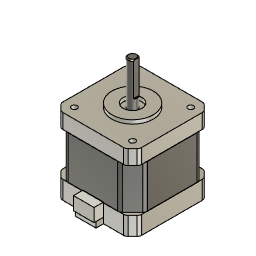
NEMA17StepperMotor (Autodesk Fusion 360 design; units mm, degrees)
Autodesk Fusion 360 part; units mm, degrees
sketch "Sketch1" plane through (0, 0, 0) normal (0, 0, 1) x (1, 0, 0)
  line L0 (-15.5, -15.5) -> (15.5, -15.5) construction
  line L1 (15.5, -15.5) -> (15.5, 15.5) construction
  line L2 (15.5, 15.5) -> (-15.5, 15.5) construction
  line L3 (-15.5, 15.5) -> (-15.5, -15.5) construction
  line L4 (0, 0) -> (0, 15.5) construction
  line L5 (0, 0) -> (15.5, 0) construction
  line L6 (-21, -21) -> (21, -21)
  line L7 (21, -21) -> (21, 21)
  line L8 (21, 21) -> (-21, 21)
  line L9 (-21, 21) -> (-21, -21)
  line L10 (-19.0919, 19.0919) -> (19.0919, -19.0919) construction
  line L11 (-21, 21) -> (21, -21) construction
  line L12 (-21, -21) -> (21, 21) construction
  line L13 (-21, 17.1838) -> (-17.1838, 21)
  line L14 (-17.1838, -21) -> (-21, -17.1838)
  line L15 (21, -17.1838) -> (17.1838, -21)
  line L16 (17.1838, 21) -> (21, 17.1838)
  dimension "d1" = 31
  dimension "d2" = 5.5
  dimension "d3" = 54
  dimension "d5" = 360
  constraint horizontal L0
  constraint vertical L1
  constraint horizontal L2
  constraint vertical L3
  constraint coincident L4.start L5.start
  constraint midpoint L1 L5.end
  constraint horizontal L5
  constraint midpoint L2 L4.end
  constraint vertical L4
  constraint equal L1 L2
  constraint coincident L4.start L10
  constraint coincident L10.end L11
  constraint coincident L10.start L11
  constraint symmetric L10.start L10.end L12
  constraint coincident L9 L13.start
  constraint coincident L8 L13.end
  constraint coincident L10.start L13
  constraint perpendicular L10 L13
  measures "d1" distance of L0.start L0.end
  measures "d3" distance of L10.start L10.end
extrude "Extrude1" add sketch "Sketch1" against normal blind 40.5 contours L6 L7 L8 L9 L13 L14 L15 L16 makes body 1
hole "Hole1" at (-15.5, -15.5, 0) direction (0, 0, -1) diameter 3 depth 6 tip angle 180 bodies 1
pattern_linear "R-Pattern1" count 2 spacing 31 along (1, 0, 0) count 2 spacing 31 along (0, 1, 0) of "Hole1"
sketch "Sketch2" plane through (0, 0, 0) normal (0, 0, 1) x (-1, 0, 0)
  circle A0 centre (-15.5, -15.5) radius 1.5
  circle A1 centre (15.5, -15.5) radius 1.5
  circle A2 centre (-15.5, 15.5) radius 1.5
  circle A3 centre (15.5, 15.5) radius 1.5
  line L0 (21, -17.1838) -> (21, 17.1838)
  line L1 (21, 17.1838) -> (17.1838, 21)
  line L2 (17.1838, 21) -> (-17.1838, 21)
  line L3 (-17.1838, 21) -> (-21, 17.1838)
  line L4 (-21, 17.1838) -> (-21, -17.1838)
  line L5 (-21, -17.1838) -> (-17.1838, -21)
  line L6 (-17.1838, -21) -> (17.1838, -21)
  line L7 (17.1838, -21) -> (21, -17.1838)
  circle A4 centre (0, 0) radius 11
  dimension "d15" = 22
  constraint coincident A4.centre origin
  measures "d15" diameter of A4
extrude "Extrude2" add sketch "Sketch2" along normal blind 2 contours A4 bodies 1
sketch "Sketch3" plane through (0, 0, 2) normal (0, 0, 1) x (-1, 0, 0)
  circle A0 centre (0, 0) radius 11
  circle A1 centre (0, 0) radius 5
  dimension "d18" = 10
  constraint coincident A0.centre A1.centre
  measures "d18" diameter of A1
extrude "Extrude3" cut sketch "Sketch3" against normal blind 2 contours A1 bodies 1
sketch "Sketch4" plane through (0, 0, 0) normal (0, 0, 1) x (-1, 0, 0)
  circle A0 centre (0, 0) radius 5
  circle A1 centre (0, 0) radius 2.5
  dimension "shaftDiameter" = 5
  constraint coincident A0.centre A1.centre
  measures "shaftDiameter" diameter of A1
extrude "Extrude4" add sketch "Sketch4" along normal blind 23.5 separate body contours A1 makes body 2
sketch "Sketch5" plane through (0, 0, 23.5) normal (0, 0, 1) x (-1, 0, 0)
  circle A0 centre (0, 0) radius 2.5
  line L0 (2.5, 0) -> (-2, 0) construction
  line L1 (-2, -1.5) -> (-2, 1.5)
  dimension "d24" = 4.5
  constraint horizontal L0
  constraint coincident A0 L0.start
  constraint coincident A0 L1.start
  constraint coincident A0 L1.end
  constraint vertical L1
  constraint coincident L0.end L1
  constraint coincident A0.centre L0
  measures "d24" distance of L0.start L0.end
chamfer "Chamfer1" distance 0.6 angle 45 1 edges at (2.3308, 0.904, 23.5) on bodies 2
extrude "Extrude5" cut sketch "Sketch5" against normal blind 18 contours A0 L1 picked at (-2.0645, 0.3999) bodies 2 1
sketch "Sketch7" plane through (0, 0, 0) normal (0, 0, 1) x (1, 0, 0)
  line L0 (-21.125, -21.125) -> (21.125, -21.125)
  line L1 (21.125, -21.125) -> (21.125, 21.125)
  line L2 (21.125, 21.125) -> (-21.125, 21.125)
  line L3 (-21.125, 21.125) -> (-21.125, -21.125)
  line L4 (-21.125, 21.125) -> (21.125, -21.125) construction
  line L5 (-21.125, -21.125) -> (21.125, 21.125) construction
  line L6 (0, 0) -> (21.125, 0) construction
  line L7 (0, 0) -> (0, 21.125) construction
  line L8 (-21.125, 14.2303) -> (-14.2303, 21.125)
  line L9 (-14.2303, -21.125) -> (-21.125, -14.2303)
  line L10 (21.125, -14.2303) -> (14.2303, -21.125)
  line L11 (14.2303, 21.125) -> (21.125, 14.2303)
  dimension "d30" = 42.25
  dimension "d31" = 25
  dimension "d33" = 360
  constraint horizontal L0
  constraint vertical L1
  constraint horizontal L2
  constraint vertical L3
  constraint equal L1 L2
  constraint coincident L6.start L4
  constraint coincident L6.start L5
  constraint coincident L6.start L7.start
  constraint midpoint L1 L6.end
  constraint midpoint L2 L7.end
  constraint coincident L3 L8.start
  constraint coincident L2 L8.end
  constraint perpendicular L4 L8
  measures "d30" distance of L1.end L2.end
  measures "d31" distance of L6.start L8
fillet "Fillet3" radius 2.5 8 edges at (-21, -17.1838, -20.25) (-17.1838, -21, -20.25) (-17.1838, 21, -20.25) (-21, 17.1838, -20.25) (17.1838, -21, -20.25) (21, -17.1838, -20.25) (21, 17.1838, -20.25) (17.1838, 21, -20.25) on bodies 1
extrude "Extrude7" cut sketch "Sketch7" against normal blind 23 from surface at -7.8 bodies 1 makes body 3 at (7, -5.3827, -30.8)
extrude "Extrude10" add sketch "Sketch7" against normal blind 23 from surface at -7.8 separate body makes body 4
extrude "Extrude6" cut sketch "Sketch7" against normal blind 23 from surface at -7.8 contours L0 L3 L9 | L0 L1 L10 | L2 L3 L8 | L1 L2 L11 bodies 4
fillet "Fillet2" radius 2.5 8 edges at (-21.125, 14.2303, -19.3) (-14.2303, 21.125, -19.3) (14.2303, 21.125, -19.3) (21.125, 14.2303, -19.3) (21.125, -14.2303, -19.3) (14.2303, -21.125, -19.3) (-14.2303, -21.125, -19.3) (-21.125, -14.2303, -19.3) on bodies 4
sketch "Sketch8" plane through (0, 0, -40.5) normal (0, 0, -1) x (1, 0, 0)
  line L0 (-21, 16.1482) -> (-21, -16.1482)
  line L1 (-20.2678, -17.916) -> (-17.916, -20.2678)
  line L2 (-16.1482, -21) -> (16.1482, -21)
  line L3 (17.916, -20.2678) -> (20.2678, -17.916)
  line L4 (21, -16.1482) -> (21, 16.1482)
  line L5 (20.2678, 17.916) -> (17.916, 20.2678)
  line L6 (16.1482, 21) -> (-16.1482, 21)
  line L7 (-17.916, 20.2678) -> (-20.2678, 17.916)
  circle A0 centre (0, 0) radius 5.1
  line L8 (-5.5, 21) -> (5.5, 21)
  line L9 (5.5, 21) -> (5.5, 25)
  line L10 (5.5, 25) -> (-5.5, 25)
  line L11 (-5.5, 25) -> (-5.5, 21)
  line L12 (0, 0) -> (0, 25) construction
  arc A1 (16.1482, -21) -> (17.916, -20.2678) centre (16.1482, -18.5) ccw
  arc A2 (20.2678, -17.916) -> (21, -16.1482) centre (18.5, -16.1482) ccw
  arc A3 (21, 16.1482) -> (20.2678, 17.916) centre (18.5, 16.1482) ccw
  arc A4 (17.916, 20.2678) -> (16.1482, 21) centre (16.1482, 18.5) ccw
  arc A5 (-16.1482, 21) -> (-17.916, 20.2678) centre (-16.1482, 18.5) ccw
  arc A6 (-20.2678, 17.916) -> (-21, 16.1482) centre (-18.5, 16.1482) ccw
  arc A7 (-21, -16.1482) -> (-20.2678, -17.916) centre (-18.5, -16.1482) ccw
  arc A8 (-17.916, -20.2678) -> (-16.1482, -21) centre (-16.1482, -18.5) ccw
  dimension "d44" = 10.2
  dimension "d45" = 4
  dimension "d46" = 11
  constraint coincident A0.centre L12.start
  constraint horizontal L8
  constraint vertical L9
  constraint horizontal L10
  constraint vertical L11
  constraint coincident L6 L8.start
  constraint midpoint L10 L12.end
  constraint vertical L12
  measures "d44" diameter of A0
  measures "d45" distance of L8.end L9.end
  measures "d46" distance of L9.end L10.end
extrude "Extrude8" add sketch "Sketch8" against normal blind 3 contours L6 L8 L9 L10 L11 bodies 2 3 1
sketch "Sketch9" plane through (0, 0, -37.5) normal (0, 0, 1) x (-1, 0, 0)
  line L0 (5.5, 21) -> (5.5, 25)
  line L1 (5.5, 25) -> (-5.5, 25)
  line L2 (-5.5, 25) -> (-5.5, 21)
  line L3 (-5.5, 21) -> (5.5, 21)
  line L4 (5.5, 25) -> (-5.5, 25)
  line L5 (-5.5, 25) -> (-5.5, 26)
  line L6 (-5.5, 26) -> (5.5, 26)
  line L7 (5.5, 26) -> (5.5, 25)
  dimension "d50" = 1
  constraint horizontal L4
  constraint vertical L5
  constraint horizontal L6
  constraint vertical L7
  constraint coincident L0.end L1.start
  constraint collinear L2 L5
  measures "d50" distance of L0.end L6.end
extrude "Extrude9" add sketch "Sketch9" along normal blind 7 separate body makes body 5
fillet "Fillet1" radius 0.2 1 edges at (2, 0, 5.5) on bodies 2
extrude "Extrude11" cut sketch "Sketch8" against normal blind 4.5 contours A0 bodies 3
equation "d2 = ( 42 mm - 31 mm ) / 2"
equation "motorheight = -40.5 mm"
equation "d19 = -( 23.5 mm - 21.5 mm )"
equation "d31 = 50 mm / 2"
equation "d51 = 10 mm - 3 mm"
